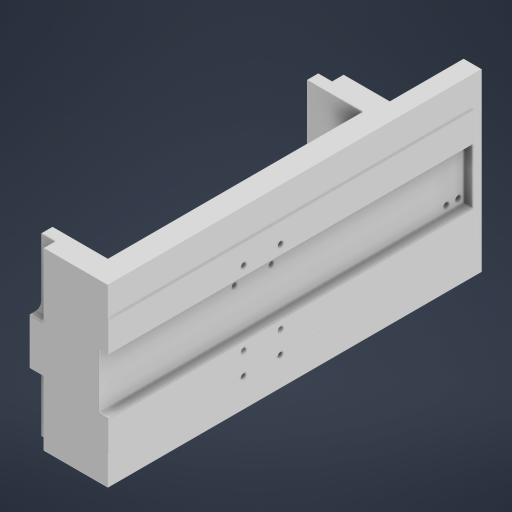
# Autodesk Inventor part: KaretkaY
Saved by Autodesk Inventor 2024 (Build 280153000, 153)
## iProperties
Created: 2023-01-08
Part Number: KaretkaY
Material: Типовые
Document SubType Name: Modeling
Designer: KirikDK
Density: 1 g/cm^3
Appearance: По умолчанию
Mass: 2127.13 g
Surface Area: 2471.04 cm^2
Volume: 2127.13 cm^3
Author: KirikDK
Autodesk Inventor part; units mm, degrees
ref_plane "YZ Plane" through (0, 0, 0) normal (1, 0, 0) x (0, 1, 0)
ref_plane "XZ Plane" through (0, 0, 0) normal (0, 1, 0) x (-1, 0, 0)
ref_plane "XY Plane" through (0, 0, 0) normal (0, 0, 1) x (1, 0, 0)
sketch "Эскиз1" plane through (0, 0, 0) normal (0, 1, 0) x (-1, 0, 0)
  line L0 (102, 151) -> (42, 151)
  line L1 (42, -149) -> (102, -149)
  line L2 (102, -149) -> (102, 151)
  line L3 (102, 151) -> (42, 151)
  line L4 (42, 151) -> (42, 176)
  line L5 (42, 176) -> (102, 176)
  line L6 (102, 176) -> (102, 151)
  line L7 (102, -149) -> (42, -149)
  line L8 (42, -149) -> (42, -124)
  line L9 (42, -124) -> (102, -124)
  line L10 (102, -124) -> (102, -149)
  line L11 (42, 176) -> (42, -124)
  line L12 (42, 176) -> (17, 176)
  line L13 (17, 176) -> (17, -149)
  line L14 (17, -149) -> (42, -149)
  line L15 (42, -149) -> (42, 176)
  point P0 (0, 0)
  point P1 (42, 151)
  dimension "d0" = 300
  dimension "d1" = 60
  dimension "d2" = 25
  dimension "d3" = 25
  dimension "d5" = 25
  dimension "d33" = 25
  constraints: 32 end point, 7 parallel, 4 horizontal, 3 perpendicular, 1 point on line
  measures "d0" distance of L1.end L0.start
  measures "d1" distance of L1.start L1.end
  measures "d2" distance between parallel lines of L0 L5
  measures "d3" distance between parallel lines of L9 L7
  measures "d5" distance between parallel lines of L15 L13
  measures "d33" distance between parallel lines of L9 L14
extrude "Выдавливание1" add sketch "Эскиз1" along normal blind 190 contours L0 L4 L5 L6 | L11 L8 L14 L13 L12 L4 | L2 L1 L8 L9
sketch "Эскиз2" plane through (-17, 0, 176) normal (1, 0, 0) x (0, 0, -1)
  line L0 (0, 0) -> (325, 0) projected
  line L1 (325, 0) -> (325, 190) projected
  line L2 (0, 190) -> (325, 190) projected
  line L3 (0, 0) -> (0, 190) projected
  line L4 (-98, 158) -> (488, 158)
  line L5 (488, 158) -> (488, 32)
  line L6 (488, 32) -> (-98, 32)
  line L7 (-98, 32) -> (-98, 158)
  point P0 (176, 0)
  point P1 (325, 32)
  point P2 (0, 32)
  point P3 (0, 158)
  point P4 (325, 158)
  dimension "d8" = 32
  dimension "d9" = 32
  constraints: 8 end point, 2 parallel, 1 horizontal, 1 perpendicular
  measures "d8" distance between parallel lines of L2 L4
  measures "d9" distance between parallel lines of L0 L6
extrude "Выдавливание2" cut sketch "Эскиз2" against normal blind 0.5 contours L3 L6 L1 L0 | L3 L2 L1 L4
sketch "Эскиз4" plane through (-102, 0, -149) normal (0, 0, -1) x (-1, 0, 0)
  line L0 (-85, 32) -> (-84.5, 32) projected
  line L1 (-84.5, 32) -> (-84.5, 0) projected
  line L2 (-84.5, 0) -> (0, 0) projected
  line L3 (0, 0) -> (0, 190) projected
  line L4 (-84.5, 190) -> (0, 190) projected
  line L5 (-84.5, 190) -> (-84.5, 158) projected
  line L6 (-84.5, 158) -> (-85, 158) projected
  line L7 (-85, 32) -> (-85, 158) projected
  line L8 (-92, 195) -> (-65, 195)
  line L9 (-65, 195) -> (-65, -10)
  line L10 (-65, -10) -> (-92, -10)
  line L11 (-92, -10) -> (-92, 195)
  point P0 (-102, 0)
  point P1 (-65, 0)
  point P2 (-65, 190)
  dimension "d12" = 20
  constraints: 8 end point, 2 parallel, 1 horizontal, 1 perpendicular
  measures "d12" distance between parallel lines of L7 L9
extrude "Выдавливание3" add sketch "Эскиз4" along normal blind 70 contours L7 L6 L5 L4 L9 L2 L1 L0
sketch "Эскиз5" plane through (-17, 32, 176) normal (1, 0, 0) x (0, 0, -1)
  line L0 (0, 0) -> (395, 0) projected
  line L1 (395, 126) -> (395, 0) projected
  line L2 (0, 126) -> (395, 126) projected
  line L3 (0, 0) -> (0, 126) projected
  line L4 (-43, 93) -> (474, 93)
  line L5 (474, 93) -> (474, 33)
  line L6 (474, 33) -> (-43, 33)
  line L7 (-43, 33) -> (-43, 93)
  point P0 (176, -32)
  dimension "d15" = 33
  dimension "d16" = 33
  constraints: 8 end point, 2 parallel, 1 horizontal, 1 perpendicular
  measures "d15" distance between parallel lines of L2 L4
  measures "d16" distance between parallel lines of L6 L0
extrude "Выдавливание4" cut sketch "Эскиз5" against normal blind 10 contours L6 L7 L4 L3 | L3 L4 L1 L6 | L1 L4 L5 L6
sketch "Эскиз6" plane through (-102, 0, -149) normal (-1, 0, 0) x (0, 0, 1)
  line L0 (0, 0) -> (25, 0) projected
  line L1 (25, 0) -> (25, 190) projected
  line L2 (0, 190) -> (25, 190) projected
  line L3 (0, 0) -> (0, 190) projected
  line L4 (300, 0) -> (325, 0) projected
  line L5 (325, 0) -> (325, 190) projected
  line L6 (300, 190) -> (325, 190) projected
  line L7 (300, 0) -> (300, 190) projected
  line L8 (325, 190) -> (-70, 190) projected
  line L9 (300, 0) -> (325, 0) projected
  line L10 (325, 190) -> (312.5, 190)
  line L11 (312.5, 190) -> (312.5, 0)
  line L12 (312.5, 0) -> (325, 0)
  line L13 (325, 0) -> (325, 190)
  line L14 (0, 190) -> (25, 190) projected
  line L15 (0, 0) -> (25, 0) projected
  line L16 (0, 190) -> (12.5, 190)
  line L17 (12.5, 190) -> (12.5, 0)
  line L18 (12.5, 0) -> (0, 0)
  line L19 (0, 0) -> (0, 190)
  line L20 (347, 70) -> (-28, 70)
  line L21 (-28, 70) -> (-28, 120)
  line L22 (-28, 120) -> (347, 120)
  line L23 (347, 120) -> (347, 70)
  point P0 (149, 0)
  point P1 (12.5, 0)
  point P2 (12.5, 190)
  point P3 (12.5, 70)
  point P4 (0, 70)
  point P5 (0, 120)
  point P6 (12.5, 120)
  point P7 (325, 70)
  point P8 (312.5, 70)
  point P9 (312.5, 120)
  point P10 (325, 120)
  dimension "d21" = 70
  dimension "d22" = 70
  constraints: 24 end point, 6 parallel, 3 horizontal, 3 perpendicular, 2 midpoint
  measures "d21" distance between parallel lines of L0 L20
  measures "d22" distance between parallel lines of L22 L2
extrude "Выдавливание5" cut sketch "Эскиз6" against normal blind 15 contours L3 L20 L17 L0 | L3 L2 L17 L22 | L20 L5 L4 L11 | L11 L6 L5 L22
fillet "Сопряжение1" radius 6 4 edges at (-94.5, 70, -136.5) (-94.5, 120, -136.5) (-94.5, 120, 163.5) (-94.5, 70, 163.5)
sketch "Эскиз8" plane through (-17, 158, 176) normal (1, 0, 0) x (0, 0, -1)
  line L0 (376, -40) -> (389, -40)
  line L1 (389, -40) -> (389, -86)
  line L2 (389, -86) -> (376, -86)
  line L3 (376, -86) -> (376, -40)
  line L4 (395, -33) -> (395, -93) projected
  circle A0 centre (389, -40) radius 3
  circle A1 centre (389, -86) radius 3
  circle A2 centre (376, -40) radius 3
  circle A3 centre (376, -86) radius 3
  point P0 (176, -158)
  dimension "d24" = 6
  dimension "d25" = 46
  dimension "d26" = 13
  constraints: 8 end point, 4 centre point, 4 coincident, 2 parallel, 1 horizontal, 1 perpendicular
  measures "d24" distance between parallel lines of L4 L1
  measures "d25" distance between parallel lines of L2 L0
  measures "d26" distance between parallel lines of L1 L3
extrude "Выдавливание6" cut sketch "Эскиз8" against normal blind 100 contours L3 A2 L0 | L0 A2 L3 | A0 L1 L0 | L0 L1 A0 | A3 L2 L3 | L3 L2 A3 | A1 L2 L1 | L1 L2 A1
sketch "Эскиз9" plane through (-102, 0, -219) normal (0, 0, -1) x (-1, 0, 0)
  line L0 (-84.5, 190) -> (-84.5, 158) projected
  line L1 (-65, 0) -> (-15, 0) projected
  line L2 (-84.5, 190) -> (-65, 190)
  line L3 (-65, 190) -> (-65, 0)
  line L4 (-65, 0) -> (-84.5, 0)
  line L5 (-84.5, 0) -> (-84.5, 190)
  point P0 (-102, 0)
  point P1 (-84.5, 158)
  constraints: 8 end point, 2 parallel, 1 horizontal, 1 perpendicular
extrude "Выдавливание7" add sketch "Эскиз9" along normal blind 10
sketch "Эскиз10" plane through (-42, 0, -124) normal (-1, 0, 0) x (0, 0, 1)
  line L0 (159.1033, 24) -> (108.1033, 24)
  line L1 (159.1033, 63) -> (159.1033, 24)
  line L2 (108.1033, 63) -> (159.1033, 63)
  line L3 (108.1033, 24) -> (108.1033, 63)
  circle A0 centre (153.6033, 31.5) radius 2.75
  circle A1 centre (113.6033, 31.5) radius 2.75
  circle A2 centre (113.6033, 55.5) radius 2.75
  circle A3 centre (153.6033, 55.5) radius 2.75
  line L4 (158.6033, 104) -> (159.6033, 104)
  line L5 (159.1033, 104) -> (159.1033, 63)
  line L6 (159.1033, 104) -> (108.1033, 104)
  line L7 (159.1033, 143) -> (159.1033, 104)
  line L8 (108.1033, 143) -> (159.1033, 143)
  line L9 (108.1033, 104) -> (108.1033, 143)
  circle A4 centre (153.6033, 111.5) radius 2.75
  circle A5 centre (113.6033, 111.5) radius 2.75
  circle A6 centre (113.6033, 135.5) radius 2.75
  circle A7 centre (153.6033, 135.5) radius 2.75
  line L10 (275, 0) -> (275, 190) projected
  line L11 (275, 26) -> (165, 26)
  line L12 (165, 26) -> (165, 46)
  line L13 (165, 46) -> (275, 46)
  line L14 (275, 46) -> (275, 26)
  line L15 (165, 26) -> (163, 26)
  line L16 (164.1033, 26) -> (164.1033, 24)
  point P0 (124, 0)
  point P1 (133.6033, 23.5)
  point P2 (133.6033, 103.5)
  constraints: 32 end point, 8 centre point, 3 horizontal, 2 parallel, 2 point on line, 2 vertical, 1 perpendicular
extrude "Выдавливание8" cut sketch "Эскиз10" against normal blind 33 contours A0 | A1 | A2 | A3 | A4 | A5 | A6 | A7
sketch "Sketch11" plane through (0, 190, 0) normal (0, 1, 0) x (1, 0, 0)
  line L0 (-42, -151) -> (-102, -151) projected
  line L1 (-102, -151) -> (-42, -151)
  line L2 (-42, -151) -> (-42, -151.5)
  line L3 (-42, -151.5) -> (-102, -151.5)
  line L4 (-102, -151.5) -> (-102, -151)
  line L5 (-102, 124) -> (-42, 124)
  line L6 (-42, 124) -> (-42, 124.5)
  line L7 (-42, 124.5) -> (-102, 124.5)
  line L8 (-102, 124.5) -> (-102, 124)
  line L9 (-17.5, -176) -> (-17.5, 229) projected
  point P0 (0, 0)
  dimension "d34" = 24.5
  dimension "d35" = 24.5
  dimension "d36" = 0.5
  dimension "d37" = 0.5
  constraints: 16 end point, 4 parallel, 2 horizontal, 2 perpendicular, 1 point on line
  measures "d34" distance between parallel lines of L9 L6
  measures "d35" distance between parallel lines of L9 L2
  measures "d36" distance between parallel lines of L0 L3
  measures "d37" distance between parallel lines of L5 L7
extrude "Extrusion9" cut sketch "Sketch11" against normal blind 200
sketch "Sketch12" plane through (-42, 0, 151.5) normal (-1, 0, 0) x (0, 0, 1)
  line L0 (-276, 190) -> (-276, 0) projected
  line L1 (-276, 80) -> (-264, 80)
  line L2 (-264, 80) -> (-264, 110)
  line L3 (-264, 110) -> (-276, 110)
  line L4 (-276, 110) -> (-276, 80)
  line L5 (0, 190) -> (0, 0) projected
  line L6 (0, 80) -> (-12, 80)
  line L7 (-12, 80) -> (-12, 110)
  line L8 (-12, 110) -> (0, 110)
  line L9 (0, 110) -> (0, 80)
  line L10 (-276, 190) -> (0, 190) projected
  line L11 (0, 0) -> (-276, 0) projected
  point P0 (-151.5, 0)
  point P1 (0, 110)
  dimension "d40" = 80
  dimension "d41" = 80
  dimension "d42" = 80
  dimension "d43" = 80
  dimension "d46" = 12
  dimension "d47" = 12
  constraints: 16 end point, 4 parallel, 2 horizontal, 2 perpendicular, 2 point on line
  measures "d40" distance between parallel lines of L10 L8
  measures "d41" distance between parallel lines of L11 L6
  measures "d42" distance between parallel lines of L10 L3
  measures "d43" distance between parallel lines of L11 L1
  measures "d46" distance of L2.end L3.end
  measures "d47" distance of L7.end L8.end
extrude "Extrusion10" add sketch "Sketch12" along normal blind 40 contours L3 L2 L1 L0 | L5 L6 L7 L8
